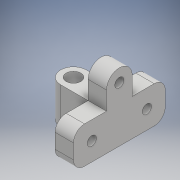
# Autodesk Inventor part: frame mount 2
Saved by Autodesk Inventor 2017 (Build 210142000, 142)
## iProperties
Created: 2017-12-13
Part Number: frame mount 2
Material: Generic
Document SubType Name: Modeling
Designer: RLanting
Density: 1 g/cm^3
Appearance: Default
Author: RLanting
Autodesk Inventor part; units mm, degrees
ref_plane "YZ Plane" through (0, 0, 0) normal (1, 0, 0) x (0, 1, 0)
ref_plane "XZ Plane" through (0, 0, 0) normal (0, 1, 0) x (-1, 0, 0)
ref_plane "XY Plane" through (0, 0, 0) normal (0, 0, 1) x (1, 0, 0)
sketch "Sketch1" plane through (0, 0, 0) normal (0, 0, 1) x (1, 0, 0)
  line L0 (0, 0) -> (-15, 0) construction
  circle A0 centre (-15, 0) radius 4
  line L1 (10, 25) -> (0, 25)
  line L2 (0, 25) -> (0, -25)
  line L3 (0, -25) -> (10, -25)
  line L4 (10, -25) -> (10, 25)
  line L5 (0, 0) -> (-15, 0) construction
  line L6 (0, 7) -> (-15, 7)
  line L7 (-15, -7) -> (0, -7)
  arc A1 (0, -7) -> (0, 7) centre (0, 0) ccw
  arc A2 (-15, 7) -> (-15, -7) centre (-15, 0) ccw
  point P0 (-7.5, 0)
  dimension "d0" = 8
  dimension "d1" = 15
  dimension "d2" = 50
  dimension "d3" = 10
  dimension "d4" = 7
  constraints: 18 end point, 4 equal length, 4 point on circle, 4 tangent, 3 centre point, 2 horizontal, 2 midpoint, 1 coincident, 1 perpendicular
  measures "d0" diameter of A0
  measures "d1" distance of L0.start L0.end
  measures "d2" distance of L1.end L2.end
  measures "d3" distance of L1.start L1.end
  measures "d4" radius of A2
extrude "Extrusion1" add sketch "Sketch1" along normal blind 20
sketch "Sketch2" plane through (10, -25, 0) normal (1, 0, 0) x (0, 0, -1)
  line L0 (0, 50) -> (-20, 50) construction
  line L1 (-10, 50) -> (-10, 40) construction
  line L2 (0, 0) -> (-20, 0) construction
  line L3 (-10, 0) -> (-10, 10) construction
  circle A0 centre (-10, 40) radius 2.5
  circle A1 centre (-10, 10) radius 2.5
  point P0 (0, 25)
  dimension "d7" = 5
  dimension "d8" = 10
  constraints: 4 end point, 2 centre point, 2 coincident, 2 midpoint, 2 vertical, 1 collinear, 1 equal radius
  measures "d7" diameter of A1
  measures "d8" distance of L3.start L3.end
extrude "Extrusion2" cut sketch "Sketch2" against normal through all
fillet "Fillet1" radius 6 4 edges at (5, 25, 20) (5, 25, 0) (5, -25, 20) (5, -25, 0)
sketch "Sketch3" plane through (10, -19, 0) normal (1, 0, 0) x (0, 0, -1)
  line L0 (-20, 15) -> (-20, 23) projected
  line L1 (-20, 19) -> (-30, 19) construction
  line L2 (-20, 26) -> (-30, 26)
  line L3 (-30, 12) -> (-20, 12)
  arc A0 (-20, 12) -> (-20, 26) centre (-20, 19) ccw
  arc A1 (-30, 26) -> (-30, 12) centre (-30, 19) ccw
  circle A2 centre (-30, 19) radius 2.5
  point P0 (0, 19)
  point P1 (-25, 19)
  dimension "d12" = 5
  dimension "d13" = 7
  dimension "d14" = 10
  constraints: 8 end point, 4 point on circle, 4 tangent, 3 centre point, 2 midpoint, 1 coincident, 1 horizontal, 1 parallel
  measures "d12" diameter of A2
  measures "d13" radius of A1
  measures "d14" distance of L1.start L1.end
extrude "Extrusion3" add sketch "Sketch3" against normal blind 10
body "Solid1"
